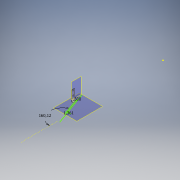
# Autodesk Inventor part: Fixação sem Tanque_2 - DIN
Saved by Autodesk Inventor 2019 (Build 230136000, 136)
## iProperties
Created: 2015-09-14
Part Number: Fixação sem Tanque_2 - DIN
Material: Genérico
Document SubType Name: Modeling
Designer: BAJA UEA
Density: 1 g/cm^3
Appearance: Padrão
Mass: 4352.78 g
Surface Area: 3520.72 cm^2
Volume: 4352.78 cm^3
Author: BAJA UEA
Autodesk Inventor part; units mm, degrees
ref_plane "YZ Plane" through (0, 0, 0) normal (1, 0, 0) x (0, 1, 0)
ref_plane "XZ Plane" through (0, 0, 0) normal (0, 1, 0) x (-1, 0, 0)
ref_plane "XY Plane" through (0, 0, 0) normal (0, 0, 1) x (1, 0, 0)
ref_plane "Plano de trabalho2" through (-1094.0332, 113.1084, -225.312) normal (0, 1, 0) x (1, 0, 0)
sketch "Esboço10" plane through (-1094.0332, 113.1084, -225.312) normal (0, 1, 0) x (1, 0, 0)
  line L0 (86.995, 81.534) -> (0, 81.534) projected
  line L1 (115.9279, -34.0424) -> (114.7048, -48.0223) projected
  line L2 (115.9279, 81.534) -> (115.9279, 81.534)
  circle A0 centre (115.9279, -5.1435) radius 8.001
  circle A1 centre (115.9279, 52.6415) radius 8.001
  line L3 (98.0571, -16.7405) -> (133.6171, -16.7405)
  line L4 (133.6171, 68.072) -> (133.6171, 42.672)
  line L5 (133.6171, -16.7405) -> (98.0571, -16.7405)
  line L6 (98.0571, -16.7405) -> (98.0571, 99.695)
  line L7 (133.6171, 99.695) -> (133.6171, -16.7405)
  line L8 (98.0571, 99.695) -> (98.0571, 110.395)
  line L9 (98.0571, 110.395) -> (133.6171, 110.395)
  line L10 (133.6171, 110.395) -> (133.6171, 99.695)
  line L11 (133.6171, 110.395) -> (98.0571, 110.395)
  line L12 (98.0571, 110.395) -> (98.0571, -16.7405)
  line L13 (98.0571, -16.7405) -> (133.6171, -16.7405)
  line L14 (133.6171, -16.7405) -> (133.6171, 110.395)
  point P0 (1094.0332, -225.312)
  point P1 (67.6228, -28.1113)
  dimension "d30" = 0
  dimension "d35" = 16.002
  dimension "d37" = 16.002
  dimension "d65" = 10.7
  constraints: 26 end point, 4 parallel, 3 horizontal, 2 centre point, 2 perpendicular
  measures "d30" distance of L2.start L2.end
  measures "d35" diameter of A0
  measures "d37" diameter of A1
  measures "d65" distance of L8.start L8.end
extrude "Extrusão9" add sketch "Esboço10" along normal blind 2
thread "Rosca1" size "11/16-12 UN" class "2B" standard "ANSI Unified Screw Threads" full length
thread "Rosca2" size "11/16-12 UN" class "2B" standard "ANSI Unified Screw Threads" full length
ref_plane "Plano de trabalho3" through (-916.6878, -44.0258, -337.707) normal (0, 0, -1) x (-1, 0, 0)
sketch "Esboço12" plane through (-916.6878, -44.0258, -337.707) normal (0, 0, -1) x (-1, 0, 0)
  line L0 (362.0216, 23.2916) -> (-61.5593, 176.4586)
  line L1 (362.0216, 44.0258) -> (812.4447, 44.0258) construction
  line L2 (209.0953, 44.0258) -> (209.0953, 78.5898)
  line L3 (26.6739, 144.5534) -> (30.9926, 156.4965)
  line L4 (30.9926, 156.4965) -> (236.8678, 82.052)
  point P0 (-916.6878, 44.0258)
  dimension "d59" = 160.12
  dimension "d63" = 34.564
  dimension "d64" = 12.7
  constraints: 10 end point, 1 coincident, 1 equal length, 1 horizontal, 1 perpendicular, 1 point on line
  measures "d59" angle of L1 L0
  measures "d63" distance of L2.start L2.end
  measures "d64" distance of L3.start L3.end
sketch "Esboço14" plane through (-960.416, 113.1084, -335.707) normal (0, 0, -1) x (-1, 0, 0)
  line L0 (-12.7356, -0.6377) -> (193.1397, -75.0822) projected
  line L1 (0, 2) -> (35.56, 2)
  line L2 (35.56, 2) -> (35.56, -18.1014)
  line L3 (0, -5.2428) -> (35.56, -18.1014)
  line L4 (0, -5.2428) -> (0, 2)
  point P0 (-960.416, -113.1084)
  constraints: 8 end point, 2 point on line, 1 collinear, 1 horizontal, 1 perpendicular, 1 vertical
extrude "Extrusão12" add sketch "Esboço14" along normal blind 2
body "Solid1"
